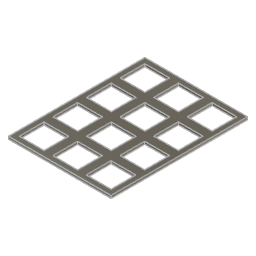
Both Models (Autodesk Fusion 360 archive; units mm, degrees)
design "Keypad Plate"
Autodesk Fusion 360 part; units mm, degrees
sketch "Sketch1" plane through (0, 0, 0) normal (0, 0, 1) x (1, 0, 0)
  line L0 (7, 7) -> (-7, 7)
  line L1 (-7, 7) -> (-7, -7)
  line L2 (-7, -7) -> (7, -7)
  line L3 (7, -7) -> (7, 7)
  line L4 (12.05, -7) -> (26.05, -7)
  line L5 (26.05, -7) -> (26.05, 7)
  line L6 (26.05, 7) -> (12.05, 7)
  line L7 (12.05, 7) -> (12.05, -7)
  line L8 (31.1, -7) -> (45.1, -7)
  line L9 (45.1, -7) -> (45.1, 7)
  line L10 (45.1, 7) -> (31.1, 7)
  line L11 (31.1, 7) -> (31.1, -7)
  line L12 (-7, -12.05) -> (7, -12.05)
  line L13 (7, -12.05) -> (7, -26.05)
  line L14 (7, -26.05) -> (-7, -26.05)
  line L15 (-7, -26.05) -> (-7, -12.05)
  line L16 (12.05, -12.05) -> (26.05, -12.05)
  line L17 (26.05, -12.05) -> (26.05, -26.05)
  line L18 (26.05, -26.05) -> (12.05, -26.05)
  line L19 (12.05, -26.05) -> (12.05, -12.05)
  line L20 (44.9974, -12.05) -> (30.9974, -12.05)
  line L21 (30.9974, -12.05) -> (30.9974, -26.05)
  line L22 (30.9974, -26.05) -> (44.9974, -26.05)
  line L23 (44.9974, -26.05) -> (44.9974, -12.05)
  line L24 (-7, -31.1) -> (7, -31.1)
  line L25 (7, -31.1) -> (7, -45.1)
  line L26 (7, -45.1) -> (-7, -45.1)
  line L27 (-7, -45.1) -> (-7, -31.1)
  line L28 (12.05, -31.1) -> (26.05, -31.1)
  line L29 (26.05, -31.1) -> (26.05, -45.1)
  line L30 (26.05, -45.1) -> (12.05, -45.1)
  line L31 (12.05, -45.1) -> (12.05, -31.1)
  line L32 (30.9974, -31.1) -> (44.9974, -31.1)
  line L33 (44.9974, -31.1) -> (44.9974, -45.1)
  line L34 (44.9974, -45.1) -> (30.9974, -45.1)
  line L35 (30.9974, -45.1) -> (30.9974, -31.1)
  line L36 (-7, -50.15) -> (7, -50.15)
  line L37 (7, -50.15) -> (7, -64.15)
  line L38 (7, -64.15) -> (-7, -64.15)
  line L39 (-7, -64.15) -> (-7, -50.15)
  line L40 (12.05, -50.15) -> (26.05, -50.15)
  line L41 (26.05, -50.15) -> (26.05, -64.15)
  line L42 (26.05, -64.15) -> (12.05, -64.15)
  line L43 (12.05, -64.15) -> (12.05, -50.15)
  line L44 (30.9974, -50.15) -> (44.9974, -50.15)
  line L45 (44.9974, -50.15) -> (44.9974, -64.15)
  line L46 (44.9974, -64.15) -> (30.9974, -64.15)
  line L47 (30.9974, -64.15) -> (30.9974, -50.15)
  line L48 (-10.05, 10.05) -> (48.0474, 10.05)
  line L49 (48.0474, 10.05) -> (48.0474, -67.2)
  line L50 (48.0474, -67.2) -> (-10.05, -67.2)
  line L51 (-10.05, -67.2) -> (-10.05, 10.05)
  point P0 (48.0474, -67.2)
  point P1 (-10.05, 10.05)
  dimension "d1" = 140
  dimension "d2" = 140
  dimension "d3" = 50.5
  dimension "d4" = 50.5
  dimension "d5" = 140
  dimension "d6" = 140
  dimension "d7" = 50.5
  dimension "d8" = 140
  dimension "d9" = 140
  dimension "d10" = 140
  dimension "d11" = 140
  dimension "d12" = 50.5
  dimension "d15" = 140
  dimension "d16" = 140
  dimension "d17" = 140
  dimension "d18" = 50.5
  dimension "d19" = 50.5
  dimension "d20" = 50.5
  dimension "d21" = 140
  dimension "d22" = 140
  dimension "d23" = 140
  dimension "d24" = 140
  dimension "d25" = 140
  dimension "d26" = 140
  dimension "d27" = 50.5
  dimension "d28" = 50.5
  dimension "d29" = 50.5
  dimension "d30" = 140
  dimension "d31" = 140
  dimension "d32" = 140
  dimension "d33" = 140
  dimension "d34" = 140
  dimension "d35" = 140
  constraint horizontal L0
  constraint perpendicular L0 L1
  constraint parallel L0 L2
  constraint parallel L1 L3
  constraint horizontal L4
  constraint vertical L5
  constraint horizontal L6
  constraint vertical L7
  constraint horizontal L8
  constraint vertical L9
  constraint horizontal L10
  constraint vertical L11
  constraint horizontal L12
  constraint vertical L13
  constraint horizontal L14
  constraint vertical L15
  constraint horizontal L16
  constraint vertical L17
  constraint horizontal L18
  constraint vertical L19
  constraint horizontal L20
  constraint vertical L21
  constraint horizontal L22
  constraint vertical L23
  constraint horizontal L24
  constraint vertical L25
  constraint horizontal L26
  constraint vertical L27
  constraint horizontal L28
  constraint vertical L29
  constraint horizontal L30
  constraint vertical L31
  constraint horizontal L32
  constraint vertical L33
  constraint horizontal L34
  constraint vertical L35
  constraint horizontal L36
  constraint vertical L37
  constraint horizontal L38
  constraint vertical L39
  constraint horizontal L40
  constraint vertical L41
  constraint horizontal L42
  constraint vertical L43
  constraint horizontal L44
  constraint vertical L45
  constraint horizontal L46
  constraint vertical L47
  constraint horizontal L48
  constraint vertical L49
  constraint horizontal L50
  constraint vertical L51
  constraint coincident P0 L49.end
  constraint coincident P1 L48.start
scale "Scale1" [no effect]
extrude "Extrude1" add sketch "Sketch1" along normal blind 1.5
